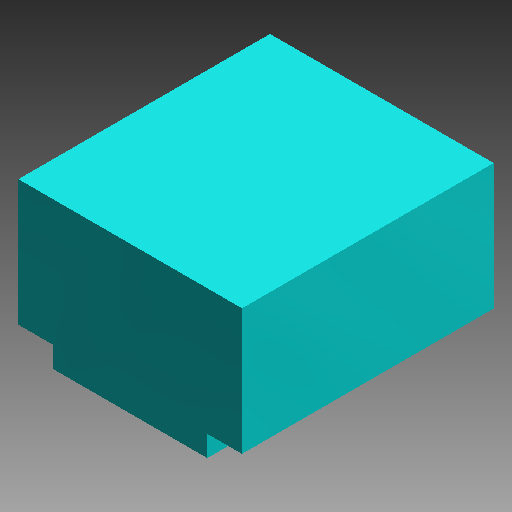
# Autodesk Inventor part: C-GRID-03-70543
Saved by Autodesk Inventor 2018.2 (Build 222227000, 227)
## iProperties
Part Number: C-GRID-03-70543
Material: Generic
Document SubType Name: Modeling
Designer: autocad
Appearance: 70543-03, C-GRID-03-70543
Author: autocad
Autodesk Inventor part; units mm, degrees
ref_plane "YZ Plane" through (0, 0, 0) normal (1, 0, 0) x (0, 1, 0)
ref_plane "XZ Plane" through (0, 0, 0) normal (0, 1, 0) x (-1, 0, 0)
ref_plane "XY Plane" through (0, 0, 0) normal (0, 0, 1) x (1, 0, 0)
sketch "70543-03, C-GRID-03-70543_93" plane through (0, 0, 0) normal (0, 0, 1) x (1, 0, 0)
  line L0 (5.0795, -2.857) -> (3.5047, -2.857)
  line L1 (3.5047, -2.857) -> (3.5047, -3.8095)
  line L2 (3.5047, -3.8095) -> (-3.492, -3.8095)
  line L3 (-3.492, -3.8095) -> (-3.492, -2.857)
  line L4 (-3.492, -2.857) -> (-5.0795, -2.857)
  line L5 (-5.0795, -2.857) -> (-5.0795, 2.8697)
  line L6 (-5.0795, 2.8697) -> (5.0795, 2.8697)
  line L7 (5.0795, 2.8697) -> (5.0795, -2.857)
  constraints: 16 end point
extrude "Extrusion1" add sketch "70543-03, C-GRID-03-70543_93" along normal blind 11.43
body "Solid1"
